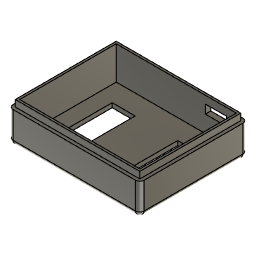
Box Coleira - Base (Autodesk Fusion 360 design; units mm, degrees)
Autodesk Fusion 360 part; units mm, degrees
sketch "Esboço1" plane through (0, 0, 0) normal (0, 0, 1) x (1, 0, 0)
  line L0 (30, 24.6) -> (-30, 24.6)
  line L1 (-30, 24.6) -> (-30, -24.6)
  line L2 (-30, -24.6) -> (30, -24.6)
  line L3 (30, -24.6) -> (30, 24.6)
  line L4 (30, 24.6) -> (-30, -24.6) construction
  line L5 (-30, 24.6) -> (30, -24.6) construction
  dimension "d1" = 60
  dimension "d2" = 49.2
  constraint horizontal L0
  constraint perpendicular L0 L1
  constraint parallel L0 L2
  constraint parallel L1 L3
  constraint coincident L4 origin
  constraint coincident L5 origin
  measures "d1" distance of L1.end L2.end
  measures "d2" distance of L0.end L1.end
extrude "Extrusão1" add sketch "Esboço1" along normal blind 14.2
sketch "Esboço2" plane through (0, 0, 14.2) normal (0, 0, 1) x (-1, 0, 0)
  line L0 (-30, 24.6) -> (-30, -24.6)
  line L1 (-30, -24.6) -> (30, -24.6)
  line L2 (30, -24.6) -> (30, 24.6)
  line L3 (30, 24.6) -> (-30, 24.6)
  line L4 (-28.5, 23.1) -> (28.5, 23.1)
  line L5 (28.5, 23.1) -> (28.5, -23.1)
  line L6 (28.5, -23.1) -> (-28.5, -23.1)
  line L7 (-28.5, -23.1) -> (-28.5, 23.1)
  line L8 (-28.5, 23.1) -> (28.5, -23.1) construction
  line L9 (28.5, 23.1) -> (-28.5, -23.1) construction
  dimension "d5" = 57
  dimension "d6" = 46.2
  constraint horizontal L4
  constraint perpendicular L4 L5
  constraint parallel L4 L6
  constraint parallel L5 L7
  constraint coincident L8 origin
  constraint coincident L9 origin
  measures "d5" distance of L5.end L6.end
  measures "d6" distance of L4.end L5.end
extrude "Extrusão2" add sketch "Esboço2" along normal blind 3 contours L4 L5 L6 L7
sketch "Esboço3" plane through (0, 0, 17.2) normal (0, 0, 1) x (-1, 0, 0)
  line L0 (-28.5, -23.1) -> (28.5, -23.1)
  line L1 (28.5, -23.1) -> (28.5, 23.1)
  line L2 (28.5, 23.1) -> (-28.5, 23.1)
  line L3 (-28.5, 23.1) -> (-28.5, -23.1)
  line L4 (-27.5, 22.1) -> (27.5, 22.1)
  line L5 (27.5, 22.1) -> (27.5, -22.1)
  line L6 (27.5, -22.1) -> (-27.5, -22.1)
  line L7 (-27.5, -22.1) -> (-27.5, 22.1)
  line L8 (-27.5, 22.1) -> (27.5, -22.1) construction
  line L9 (27.5, 22.1) -> (-27.5, -22.1) construction
  dimension "d9" = 55
  dimension "d10" = 44.2
  constraint horizontal L4
  constraint perpendicular L4 L5
  constraint parallel L4 L6
  constraint parallel L5 L7
  constraint coincident L8 origin
  constraint coincident L9 origin
  measures "d9" distance of L5.end L6.end
  measures "d10" distance of L4.end L5.end
extrude "Extrusão3" cut sketch "Esboço3" against normal blind 15.2 contours L4 L5 L6 L7
fillet "Arredondamento1" radius 2 4 edges at (-30, -24.6, 7.1) (-30, 24.6, 7.1) (30, -24.6, 7.1) (30, 24.6, 7.1)
sketch "Esboço5" plane through (30, 0, 0) normal (1, 0, 0) x (0, 1, 0)
  line L0 (22.6, 0) -> (22.6, 10)
  line L1 (22.6, 10) -> (-22.6, 10)
  line L2 (-22.6, 10) -> (-22.6, 0)
  line L3 (-22.6, 0) -> (22.6, 0)
  line L4 (15, 5.5) -> (-15, 5.5)
  line L5 (-15, 5.5) -> (-15, 8.5)
  line L6 (-15, 8.5) -> (15, 8.5)
  line L7 (15, 8.5) -> (15, 5.5)
  line L8 (15, 5.5) -> (-15, 8.5) construction
  line L9 (-15, 5.5) -> (15, 8.5) construction
  arc A0 (15, 5.5) -> (15, 8.5) centre (15, 7) ccw
  arc A1 (-15, 8.5) -> (-15, 5.5) centre (-15, 7) ccw
  point P0 (0, 7)
  dimension "d22" = 30
  dimension "d23" = 3
  constraint horizontal L4
  constraint perpendicular L4 L5
  constraint parallel L4 L6
  constraint parallel L5 L7
  constraint coincident L8 P0
  constraint coincident L9 P0
  constraint tangent L6 A0
  constraint tangent L6 A1
  measures "d22" distance of L5.end L6.end
  measures "d23" distance of L4.end L5.end
extrude "Extrusão5" [suppressed]
sketch "Esboço6" plane through (-30, 0, 0) normal (-1, 0, 0) x (0, -1, 0)
  line L0 (-22.6, 14.2) -> (-22.6, 0)
  line L1 (-22.6, 0) -> (22.6, 0)
  line L2 (22.6, 0) -> (22.6, 14.2)
  line L3 (22.6, 14.2) -> (-22.6, 14.2)
  line L4 (13.4422, 4.9877) -> (8.4422, 4.9877)
  line L5 (8.4422, 4.9877) -> (8.4422, 1.9977)
  line L6 (8.4422, 1.9977) -> (13.4422, 1.9977)
  line L7 (13.4422, 1.9977) -> (13.4422, 4.9877)
  line L8 (13.4422, 4.9877) -> (8.4422, 1.9977) construction
  line L9 (8.4422, 4.9877) -> (13.4422, 1.9977) construction
  point P0 (10.9422, 3.4927)
  dimension "d28" = 5
  dimension "d29" = 2.99
  constraint horizontal L4
  constraint perpendicular L4 L5
  constraint parallel L4 L6
  constraint parallel L5 L7
  constraint coincident L8 P0
  constraint coincident L9 P0
  measures "d28" distance of L5.end L6.end
  measures "d29" distance of L4.end L5.end
fillet "Arredondamento3" radius 2 8 edges at (0, 24.6, 0) (-29.4142, 24.0142, 0) (-30, 0, 0) (-29.4142, -24.0142, 0) (0, -24.6, 0) (29.4142, -24.0142, 0) (30, 0, 0) (29.4142, 24.0142, 0)
extrude "Extrusão8" [suppressed]
sketch "Esboço8" plane through (0, 22.1, 0) normal (0, -1, 0) x (1, 0, 0)
  line L0 (27.5, 17.2) -> (-27.5, 17.2)
  line L1 (-27.5, 17.2) -> (-27.5, 2)
  line L2 (-27.5, 2) -> (27.5, 2)
  line L3 (27.5, 2) -> (27.5, 17.2)
  line L4 (22.9733, 5.5) -> (22.9733, 9.5)
  line L5 (13.3, 9.5) -> (22.9733, 9.5)
  line L6 (22.9733, 9.5) -> (22.9733, 5.5)
  line L7 (22.9733, 5.5) -> (13.3, 5.5)
  line L8 (13.3, 5.5) -> (13.3, 9.5)
  line L9 (22.9733, 2) -> (22.9733, 9.7)
  line L10 (22.9733, 9.7) -> (13.3, 9.7)
  line L11 (13.3, 9.7) -> (13.3, 13.7)
  line L12 (13.3, 13.7) -> (22.9733, 13.7)
  line L13 (22.9733, 13.7) -> (22.9733, 9.7)
  point P0 (13.3, 8)
  dimension "d64" = 4
  dimension "d76" = 7.7
  dimension "d77" = 4
  constraint horizontal L5
  constraint vertical L6
  constraint horizontal L7
  constraint vertical L8
  constraint coincident L2 L9.start
  constraint perpendicular L7 L9
  constraint perpendicular L8 L10
  constraint perpendicular L10 L11
  constraint perpendicular L9 L12
  constraint perpendicular L10 L13
  measures "d64" distance of L5.start L7.end
  measures "d76" distance of L9.start L9.end
  measures "d77" distance of L10.end L11.end
extrude "Extrusão11" [suppressed]
sketch "Esboço9" plane through (0, 0, 2) normal (0, 0, 1) x (-1, 0, 0)
  line L0 (-27.5, -22.1) -> (27.5, -22.1)
  line L1 (27.5, -22.1) -> (27.5, 22.1)
  line L2 (27.5, 22.1) -> (-27.5, 22.1)
  line L3 (-27.5, 22.1) -> (-27.5, -22.1)
  line L4 (9.75, -13) -> (20.25, -13)
  line L5 (20.25, -13) -> (20.25, 13)
  line L6 (20.25, 13) -> (9.75, 13)
  line L7 (9.75, 13) -> (9.75, -13)
  line L8 (9.75, -13) -> (20.25, 13) construction
  line L9 (20.25, -13) -> (9.75, 13) construction
  line L10 (-9.75, -13) -> (-20.25, -13)
  line L11 (-20.25, -13) -> (-20.25, 13)
  line L12 (-20.25, 13) -> (-9.75, 13)
  line L13 (-9.75, 13) -> (-9.75, -13)
  line L14 (-9.75, -13) -> (-20.25, 13) construction
  line L15 (-20.25, -13) -> (-9.75, 13) construction
  point P0 (15, 0)
  point P1 (-15, 0)
  dimension "d68" = 10.5
  dimension "d69" = 26
  dimension "d72" = 10.5
  dimension "d73" = 26
  constraint horizontal L4
  constraint perpendicular L4 L5
  constraint parallel L4 L6
  constraint parallel L5 L7
  constraint coincident L8 P0
  constraint coincident L9 P0
  constraint horizontal L10
  constraint perpendicular L10 L11
  constraint parallel L10 L12
  constraint parallel L11 L13
  constraint coincident L14 P1
  constraint coincident L15 P1
  measures "d68" distance of L5.end L6.end
  measures "d69" distance of L4.end L5.end
  measures "d72" distance of L11.end L12.end
  measures "d73" distance of L10.end L11.end
extrude "Extrusão12" cut sketch "Esboço9" against normal blind 2 contours L4 L5 L6 L7 | L10 L11 L12 L13
extrude "Extrusão13" cut sketch "Esboço8" against normal blind 3.5 contours L10 L11 L12 L13
